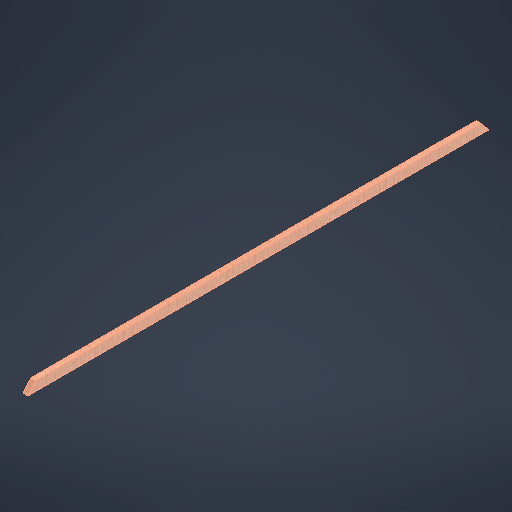
# Autodesk Inventor part: BASE_SIDEK_TREBUCHET
Saved by Autodesk Inventor 2026.2 (Build 302298010, 298A)
## iProperties
Created: 2026-02-18
Part Number: BASE_SIDEK_TREBUCHET
Material: Wood (Oak)
Document SubType Name: Modeling
Designer: 4aida
Density: 0.76 g/cm^3
Appearance: White Oak - Natural Medium Gloss
Mass: 176.907 g
Surface Area: 869.907 cm^2
Volume: 232.772 cm^3
Author: 4aida
Autodesk Inventor part; units mm, degrees
ref_plane "YZ Plane" through (0, 0, 0) normal (1, 0, 0) x (0, 1, 0)
ref_plane "XZ Plane" through (0, 0, 0) normal (0, 1, 0) x (-1, 0, 0)
ref_plane "XY Plane" through (0, 0, 0) normal (0, 0, 1) x (1, 0, 0)
sketch "Sketch1" plane through (0, 0, 0) normal (1, 0, 0) x (0, 1, 0)
  line L0 (-9.1281, -447.675) -> (9.1281, -447.675) construction
  line L1 (9.1281, -447.675) -> (9.1281, 447.675)
  line L2 (9.1281, 447.675) -> (-9.1281, 447.675) construction
  line L3 (-9.1281, 447.675) -> (-9.1281, -447.675)
  line L4 (-9.1281, -447.675) -> (9.1281, 447.675) construction
  line L5 (9.1281, -447.675) -> (-9.1281, 447.675) construction
  line L6 (-9.1281, 447.675) -> (9.1281, 432.3562)
  line L7 (-9.1281, -447.675) -> (9.1281, -432.3562)
  point P0 (0, 0)
  dimension "d0" = 895.35
  dimension "d1" = 18.2563
  dimension "d16" = 40
  dimension "d17" = 40
  constraints: 16 end point, 2 midpoint, 2 parallel, 2 point on line, 1 horizontal, 1 perpendicular
  measures "d0" distance of L0.end L1.end
  measures "d1" distance of L1.end L2.end
  measures "d16" angle of L2 L6
  measures "d17" angle of L7 L0
extrude "Extrusion1" add sketch "Sketch1" along normal blind 9.525
body "Solid1"
